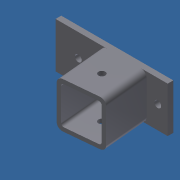
# Autodesk Inventor part: frame bracket
Saved by Autodesk Inventor 2012 (Build 160160000, 160)
## iProperties
Created: 2012-03-08
Part Number: frame bracket
Material: Steel
Document SubType Name: Modeling
Designer: esv
Mass: 714.408 g
Surface Area: 337.789 cm^2
Volume: 81.4684 cm^3
Density: 8.76914 g/cm^3
Author: esv
Autodesk Inventor part; units mm, degrees
ref_plane "YZ Plane" through (0, 0, 0) normal (1, 0, 0) x (0, 1, 0)
ref_plane "XZ Plane" through (0, 0, 0) normal (0, 1, 0) x (-1, 0, 0)
ref_plane "XY Plane" through (0, 0, 0) normal (0, 0, 1) x (1, 0, 0)
sketch "Sketch1" plane through (0, 0, 0) normal (0, 0, 1) x (1, 0, 0)
  line L0 (0, 0) -> (125.4125, 0)
  line L1 (125.4125, 0) -> (125.4125, 50.8)
  line L2 (125.4125, 50.8) -> (0, 50.8)
  line L3 (0, 50.8) -> (0, 0)
  dimension "d0" = 50.8
  dimension "d1" = 125.4125
  constraints: 8 end point, 2 parallel, 1 coincident, 1 horizontal, 1 perpendicular
  measures "d0" distance of L2.end L0.start
  measures "d1" distance of L0.start L0.end
extrude "Extrusion1" add sketch "Sketch1" along normal blind 6.35
sketch "Sketch2" plane through (0, 0, 6.35) normal (0, 0, 1) x (1, 0, 0)
  line L0 (0, 0) -> (0, 50.8) projected
  line L1 (125.4125, 50.8) -> (125.4125, 0) projected
  point P0 (25.4, 25.4)
  point P1 (114.3, 25.4)
  point P2 (0, 25.4)
  dimension "d4" = 25.4
  dimension "d5" = 11.1125
  constraints: 2 horizontal alignment, 1 midpoint
  measures "d4" distance from line of L0 point (25.4, 25.4)
  measures "d5" distance from line of L1 point (114.3, 25.4)
hole "Hole1" at (25.4, 25.4, 6.35) at (114.3, 25.4, 6.35) direction (0, 0, -1) diameter 7.62 end through all
sketch "Sketch3" plane through (0, 50.8, 0) normal (0, 1, 0) x (1, 0, 0)
  line L0 (0, -6.35) -> (125.4125, -6.35) projected
  line L1 (0, 0) -> (0, -6.35) projected
  line L2 (101.8247, -6.35) -> (106.5326, -56.3502)
  line L3 (106.5326, -56.3502) -> (55.9563, -61.1124)
  line L4 (55.9563, -61.1124) -> (50.8, -6.35)
  dimension "d13" = 50.8
  dimension "d14" = 50.8
  dimension "d15" = 54.7624
  dimension "d16" = 5.379
  constraints: 6 end point, 2 point on line, 1 parallel, 1 perpendicular
  measures "d13" distance between parallel lines of L4 L2
  measures "d14" distance from line of L4.end L1
  measures "d15" distance from line of L0 L3.end
  measures "d16" angle of L1 L4
extrude "Extrusion2" add sketch "Sketch3" against normal up to surface (50.8 mm away)
sketch "Sketch4" plane through (106.5326, 0, 56.3502) normal (0.0937434, 0, 0.9955964) x (0.9955964, 0, -0.0937434)
  line L0 (-50.8, 50.8) -> (0, 50.8) projected
  line L1 (-50.8, 50.8) -> (-50.8, 0) projected
  line L2 (-43.18, 46.355) -> (-7.62, 46.355)
  line L3 (-4.445, 43.18) -> (-4.445, 7.62)
  line L4 (-7.62, 4.445) -> (-43.18, 4.445)
  line L5 (-46.355, 7.62) -> (-46.355, 43.18)
  arc A0 (-43.18, 46.355) -> (-46.355, 43.18) centre (-43.18, 43.18) ccw
  arc A1 (-46.355, 7.62) -> (-43.18, 4.445) centre (-43.18, 7.62) ccw
  arc A2 (-7.62, 4.445) -> (-4.445, 7.62) centre (-7.62, 7.62) ccw
  arc A3 (-4.445, 43.18) -> (-7.62, 46.355) centre (-7.62, 43.18) ccw
  point P0 (-100.781, 0)
  point P1 (-25.4, 46.355)
  point P2 (-25.4, 50.8)
  point P3 (-46.355, 25.4)
  point P4 (-50.8, 25.4)
  dimension "d19" = 3.175
  dimension "d20" = 4.445
  dimension "d21" = 4.445
  constraints: 8 end point, 8 point on circle, 8 tangent, 4 centre point, 4 midpoint, 3 equal radius, 2 parallel, 1 horizontal, 1 horizontal alignment, 1 perpendicular, 1 vertical alignment
  measures "d19" radius of A0
  measures "d20" distance between parallel lines of L1 L5
  measures "d21" distance between parallel lines of L0 L2
extrude "Extrusion3" cut sketch "Sketch4" against normal up to surface surface through (62.7063, 25.4, 6.35) normal (0, 0, 1)
fillet "Fillet1" radius 6.35 4 edges at (53.3782, 50.8, 33.7312) (53.3782, 0, 33.7312) (104.1787, 50.8, 31.3501) (104.1787, 0, 31.3501)
hole "Hole2" at (78.8634, 50.8, 33.4432) direction (0, -1, 0) diameter 7.62 end through all
body "Solid1"
